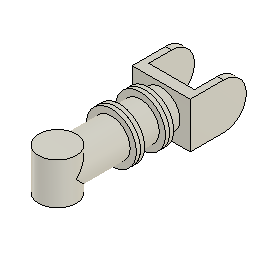
trail_link2 (Autodesk Fusion 360 design; units mm, degrees)
Autodesk Fusion 360 part; units mm, degrees
note: some values were not read from the file. Set by a fixed rule: which sketch regions a step uses.
sketch "Sketch1" plane through (0, 0, 0) normal (0, 1, 0) x (1, 0, 0)
  circle A0 centre (0, 0) radius 45
  circle A1 centre (0, 0) radius 30
  dimension "d1" = 90
  constraint coincident A0.centre A1.centre
  measures "d1" diameter of A0
extrude "Extrude1" add sketch "Sketch1" along normal blind 50 makes body 1
sketch "Sketch2" plane through (0, 0, 0) normal (0, -1, 0) x (1, 0, 0)
  circle A0 centre (0, 0) radius 30
  circle A1 centre (0, 0) radius 45
  circle A2 centre (0, 0) radius 60
  constraint coincident A0.centre A1.centre
extrude "Extrude2" add sketch "Sketch2" along normal blind 10 separate body contours A1 | A2 makes body 2
sketch "Sketch3" plane through (0, -10, 0) normal (0, -1, 0) x (1, 0, 0)
  circle A0 centre (0, 0) radius 30
  circle A1 centre (0, 0) radius 60
  line L0 (0, 0) -> (80, 0) construction
copy_body "CopyPasteBodies1" bodies 2 makes body 3
move_body "Move1" bodies 3 to x (1, 0, 0) y (0, 1, 0) z (0, 0, 1) at (0, 60, 0)
copy_body "CopyPasteBodies2" bodies 2 makes body 4
move_body "Move2" bodies 4 to x (1, 0, 0) y (0, 1, 0) z (0, 0, 1) at (0, -10, 0)
sketch "Sketch7" plane through (0, 0, 0) normal (0, 0, 1) x (1, 0, 0)
  line L0 (0, -20) -> (0, -150) construction
  circle A0 centre (0, -150) radius 45
  dimension "d17" = 130
  dimension "d18" = 90
  constraint vertical L0
  constraint coincident L0.end A0.centre
  measures "d17" distance of L0.start L0.end
  measures "d18" diameter of A0
extrude "Extrude5" add sketch "Sketch7" along normal mid plane 100 separate body makes body 5
sketch "Sketch8" plane through (0, -20, 0) normal (0, -1, 0) x (1, 0, 0)
  circle A0 centre (0, 0) radius 30
  circle A1 centre (0, 0) radius 60
  circle A2 centre (0, 0) radius 45
  dimension "d21" = 90
  constraint coincident A0.centre A1.centre
  measures "d21" diameter of A2
extrude "Extrude6" add sketch "Sketch8" along normal blind 130 contours A2 bodies 5 4
sketch "Sketch9" plane through (0, 0, 50) normal (0, 0, 1) x (-1, 0, 0)
  circle A0 centre (0, 150) radius 45
copy_body "CopyPasteBodies3" bodies 3 makes body 6
move_body "Move3" bodies 6 to x (1, 0, 0) y (0, 1, 0) z (0, 0, 1) at (0, 10, 0)
sketch "Sketch10" plane through (0, 70, 0) normal (0, 1, 0) x (-1, 0, 0)
  circle A0 centre (0, 0) radius 30
  circle A1 centre (0, 0) radius 60
  circle A2 centre (0, 0) radius 45
  dimension "d26" = 90
  constraint coincident A0.centre A1.centre
  measures "d26" diameter of A2
extrude "Extrude8" add sketch "Sketch10" along normal blind 30 contours A2 bodies 6
sketch "Sketch12" plane through (0, 0, 0) normal (1, 0, 0) x (0, 1, 0)
  line L0 (100, 0) -> (100, 55)
  line L1 (100, 0) -> (100, -55)
  line L2 (100, 55) -> (180, 55)
  line L3 (100, -55) -> (180, -55)
  arc A0 (180, -55) -> (180, 55) centre (180, 0) ccw
  dimension "d38" = 55
  dimension "d39" = 55
  dimension "d40" = 80
  constraint vertical L0
  constraint parallel L0 L1
  constraint perpendicular L0 L2
  constraint perpendicular L1 L3
  constraint tangent L3 A0
  measures "d38" distance of L0.start L0.end
  measures "d39" distance of L0.start L1.end
  measures "d40" distance of L0.end L2.end
extrude "Extrude10" add sketch "Sketch12" along normal mid plane 140 bodies 6
ref_plane "WorkPlane1" through (-10.8818, 235, 0) normal (0, 1, 0) x (0, 0, -1)
sketch "Sketch13" plane through (-10.8818, 235, 0) normal (0, 1, 0) x (1, 0, 0)
  line L0 (65.8818, -123.2975) -> (-44.1182, -123.2975)
  line L1 (-44.1182, -123.2975) -> (-44.1182, 110)
  line L2 (-44.1182, 110) -> (65.8818, 110)
  line L3 (65.8818, 110) -> (65.8818, -123.2975)
  line L4 (-59.1182, 55) -> (-59.1182, -55)
  line L5 (80.8818, -55) -> (80.8818, 55)
  dimension "d44" = 15
  dimension "d45" = 15
  constraint horizontal L0
  constraint vertical L1
  constraint horizontal L2
  constraint vertical L3
  measures "d44" distance of L1 L4
  measures "d45" distance of L3 L5
extrude "Extrude11" cut sketch "Sketch13" against normal blind 110 bodies 6
sketch "Sketch14" plane through (70, 0, 0) normal (1, 0, 0) x (0, 1, 0)
  line L0 (100, 55) -> (100, -55)
  line L1 (100, -55) -> (180, -55)
  arc A0 (180, -55) -> (180, 55) centre (180, 0) ccw
  line L2 (180, 55) -> (100, 55)
  line L3 (180, 0) -> (219.0512, 0) construction
  constraint horizontal L3
scale "Scale1" factor 0.5 about (-30, 50, 0) bodies 6 5 1 2 3
extrude "Extrude12" [rolled back] along distance -50 taper angle 0
ref_plane "WorkPlane2" through (45, -150, 15.2069) normal (1, 0, 0) x (0, -1, 0)
sketch "Sketch16" plane through (0, 0, 0) normal (1, 0, 0) x (0, 1, 0)
  line L0 (-155, 35) -> (-155, 15)
  arc A0 (-155, 15) -> (-145, 15) centre (-150, 15) ccw
  line L1 (-145, 15) -> (-145, 35)
  arc A1 (-145, 35) -> (-155, 35) centre (-150, 35) ccw
  line L2 (-150, 35) -> (-150, 15) construction
  line L3 (-155, -15) -> (-155, -35)
  arc A2 (-155, -35) -> (-145, -35) centre (-150, -35) ccw
  line L4 (-145, -35) -> (-145, -15)
  arc A3 (-145, -15) -> (-155, -15) centre (-150, -15) ccw
  line L5 (-150, -15) -> (-150, -35) construction
  point P0 (-150, 50)
  point P1 (-150, -50)
  dimension "d65" = 10
  dimension "d66" = 10
  dimension "d67" = 20
  dimension "d68" = 20
  dimension "d69" = 30
  dimension "d70" = 15
  dimension "d71" = 15
  constraint tangent L0 A0
  constraint tangent A0 L1
  constraint parallel L0 L1
  constraint tangent L1 A1
  constraint tangent L0 A1
  constraint vertical L2
  constraint tangent L3 A2
  constraint tangent A2 L4
  constraint parallel L3 L4
  constraint tangent L4 A3
  constraint tangent L3 A3
  constraint parallel L2 L5
  measures "d65" diameter of A0
  measures "d66" diameter of A2
  measures "d67" distance of A3.centre A2.centre
  measures "d68" distance of A1.centre A0.centre
  measures "d69" distance of A0.centre A3.centre
  measures "d70" distance of A1.centre P0
  measures "d71" distance of A2.centre P1
extrude "Extrude14" [rolled back] along distance 70 taper angle 0
